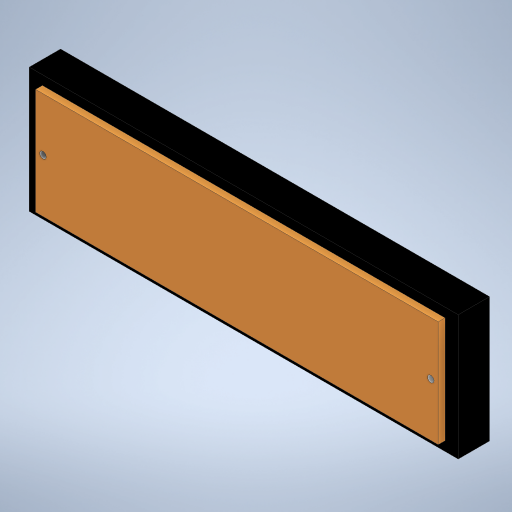
# Autodesk Inventor part: TH22_soroban_sn
Saved by Autodesk Inventor 2023 (Build 270158000, 158)
## iProperties
Created: 2021-10-06
Part Number: TH22_soroban_sn
Material: ABS プラスチック
Document SubType Name: Modeling
Designer: 中島 青蔵
Density: 1.06 g/cm^3
Appearance: 滑らか - 白
Author: 中島 青蔵
Autodesk Inventor part; units mm, degrees
ref_plane "YZ Plane" through (0, 0, 0) normal (1, 0, 0) x (0, 1, 0)
ref_plane "XZ Plane" through (0, 0, 0) normal (0, 1, 0) x (-1, 0, 0)
ref_plane "XY Plane" through (0, 0, 0) normal (0, 0, 1) x (1, 0, 0)
sketch "スケッチ1" plane through (0, 0, 0) normal (0, 0, 1) x (1, 0, 0)
  line L0 (0, 0) -> (208, 0)
  line L1 (208, 0) -> (208, 60.6)
  line L2 (208, 60.6) -> (0, 60.6)
  line L3 (0, 60.6) -> (0, 0)
  line L4 (6.4, 4.5) -> (201.6, 4.5)
  line L5 (201.6, 4.5) -> (201.6, 56.1)
  line L6 (201.6, 56.1) -> (6.4, 56.1)
  line L7 (6.4, 56.1) -> (6.4, 4.5)
  dimension "d0" = 208
  dimension "d1" = 60.6
  dimension "d2" = 195.2
  dimension "d3" = 51.6
  constraints: 16 end point
  measures "d0" distance of L2.end L1.end
  measures "d1" distance of L1.end L0.end
  measures "d2" distance of L6.end L5.end
  measures "d3" distance of L5.end L4.end
extrude "押し出し1" add sketch "スケッチ1" along normal blind 15.2
extrude "押し出し2" add sketch "スケッチ1" along normal blind 18.5 contours L7 L6 L5 L4
sketch "スケッチ2" plane through (0, 0, 0) normal (0, 0, -1) x (-1, 0, 0)
  line L0 (0, 60.6) -> (0, 0) projected
  line L1 (-208, 0) -> (-208, 60.6) projected
  line L2 (0, 0) -> (-208, 0) projected
  point P0 (-198, 30.3)
  point P1 (-10, 30.3)
  dimension "d8" = 10
  dimension "d9" = 10
  dimension "d19" = 30.3
  dimension "d22" = 30.3
  measures "d8" distance from line of L0 point (-10, 30.3)
  measures "d9" distance from line of L1 point (-198, 30.3)
  measures "d19" distance from line of L2 point (-10, 30.3)
  measures "d22" distance from line of L2 point (-198, 30.3)
hole "穴1" at (198, 30.3, 0) at (10, 30.3, 0) direction (0, 0, 1) diameter 3.2 end through all
equation "\"d19\" = d22"
